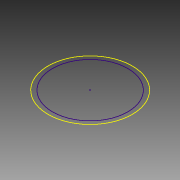
# Autodesk Inventor part: PSteg
Saved by Autodesk Inventor 2014 (Build 180170000, 170)
## iProperties
Created: 2013-05-23
Part Number: PSteg
Material: Generisch
Document SubType Name: Modeling
Designer: hartmann
Density: 1 g/cm^3
Appearance: Vorgabe
Author: hartmann
Autodesk Inventor part; units mm, degrees
ref_plane "YZ Plane" through (0, 0, 0) normal (1, 0, 0) x (0, 1, 0)
ref_plane "XZ Plane" through (0, 0, 0) normal (0, 1, 0) x (-1, 0, 0)
ref_plane "XY Plane" through (0, 0, 0) normal (0, 0, 1) x (1, 0, 0)
sketch "Skizze4" plane through (0, 0, 0) normal (0, 0, 1) x (1, 0, 0)
  circle A0 centre (0, 0) radius 9.1575 projected
  circle A1 centre (0, 0) radius 10.6575 projected
  circle A2 centre (0, 0) radius 9.1575
  constraints: 1 centre point, 1 coincident, 1 concentric
extrude "Extrusion3" add sketch "Skizze4" along normal blind 2 contours A0
sketch "Skizze5" plane through (0, 0, 0) normal (0, 0, -1) x (-1, 0, 0)
  circle A0 centre (-2.1708, 6.2328) radius 1.5 projected
  circle A1 centre (-4.3123, -4.9964) radius 1.5 projected
  circle A2 centre (6.4832, -1.2364) radius 1.5 projected
extrude "Extrusion4" add sketch "Skizze5" along normal blind 2
